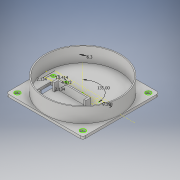
# Autodesk Inventor part: Bottom Sensor Base v1.3
Saved by Autodesk Inventor 2019 (Build 230136000, 136)
## iProperties
Created: 2020-01-12
Part Number: Bottom Sensor Base v1.3
Material: Generic
Document SubType Name: Modeling
Designer: Obscure_Decision
Density: 1 g/cm^3
Appearance: Default
Author: Obscure_Decision
Autodesk Inventor part; units mm, degrees
ref_plane "YZ Plane" through (0, 0, 0) normal (1, 0, 0) x (0, 1, 0)
ref_plane "XZ Plane" through (0, 0, 0) normal (0, 1, 0) x (-1, 0, 0)
ref_plane "XY Plane" through (0, 0, 0) normal (0, 0, 1) x (1, 0, 0)
sketch "Bottom" plane through (0, 0, 0) normal (0, 0, 1) x (1, 0, 0)
  line L0 (0, 0) -> (88.9, 0)
  line L1 (88.9, 0) -> (88.9, -3.0988)
  line L2 (88.9, -3.0988) -> (0, -3.0988)
  line L3 (0, -3.0988) -> (0, 0)
  line L4 (44.45, -3.0988) -> (44.45, 0)
  line L5 (44.45, 0) -> (90.932, 0)
  line L6 (44.45, 0) -> (90.932, 0)
  line L7 (90.932, 0) -> (90.932, -3.0988)
  line L8 (90.932, -3.0988) -> (44.45, -3.0988)
  line L9 (44.45, -3.0988) -> (44.45, 0)
  line L10 (44.45, 0) -> (-2.032, 0)
  line L11 (-2.032, 0) -> (-2.032, -3.0988)
  line L12 (-2.032, -3.0988) -> (44.45, -3.0988)
  line L13 (44.45, -3.0988) -> (44.45, 0)
  dimension "d0" = 88.9
  dimension "d1" = 3.0988
  dimension "d3" = 46.482
  dimension "d4" = 46.482
  constraints: 28 end point, 6 parallel, 4 horizontal, 3 perpendicular, 2 midpoint
  measures "d0" distance of L1.end L2.end
  measures "d1" distance of L0.end L1.end
  measures "d3" distance of L7.end L8.end
  measures "d4" distance of L11.end L12.end
revolve "Bottom Base" add sketch "Bottom" angle 360 about axis through (44.45, -3.0988, 0) along (0, 1, 0)
sketch "Outer Wall Circles" plane through (44.45, 0, 0) normal (0, 1, 0) x (1, 0, 0)
  circle A0 centre (0, 0) radius 44.45
  circle A1 centre (0, 0) radius 45.72
  point P0 (-44.45, 0)
  dimension "d6" = 88.9
  dimension "d77" = 91.44
  constraints: 2 centre point, 1 coincident
  measures "d6" diameter of A0
  measures "d77" diameter of A1
extrude "Outer Wall Extr" add sketch "Outer Wall Circles" along normal blind 17.78
sketch "Mount Square" plane through (44.45, -3.0988, 0) normal (0, -1, 0) x (1, 0, 0)
  circle A0 centre (0, 0) radius 46.482
  line L0 (43.307, -46.482) -> (-43.307, -46.482)
  line L1 (-46.482, -43.307) -> (-46.482, 43.307)
  line L2 (-43.307, 46.482) -> (43.307, 46.482)
  line L3 (46.482, 43.307) -> (46.482, -43.307)
  line L4 (46.482, -46.482) -> (-46.482, 46.482) construction
  line L5 (-46.482, -46.482) -> (46.482, 46.482) construction
  arc A1 (-46.482, -43.307) -> (-43.307, -46.482) centre (-43.307, -43.307) ccw
  arc A2 (43.307, -46.482) -> (46.482, -43.307) centre (43.307, -43.307) ccw
  arc A3 (46.482, 43.307) -> (43.307, 46.482) centre (43.307, 43.307) ccw
  arc A4 (-43.307, 46.482) -> (-46.482, 43.307) centre (-43.307, 43.307) ccw
  point P0 (-44.45, 0)
  dimension "d30" = 3.175
  constraints: 12 end point, 8 point on circle, 8 point on line, 8 tangent, 5 centre point, 3 equal radius, 2 midpoint, 2 parallel, 1 horizontal, 1 perpendicular
  measures "d30" radius of A1
extrude "Base Mount" add sketch "Mount Square" against normal blind 3.0988 contours L3 A2 L0 A0 | A0 L2 A3 L3 | A0 L1 A4 L2 | L0 A1 L1 A0
sketch "Silicon Circles" plane through (1.143, -3.0988, 46.482) normal (0, -1, 0) x (1, 0, 0)
  line L0 (89.789, -3.175) -> (89.789, -89.789) projected
  circle A0 centre (43.1405, -46.482) radius 44.45
  circle A1 centre (43.1405, -46.482) radius 43.18
  point P0 (-1.143, -46.482)
  dimension "d37" = 88.9
  dimension "d38" = 86.36
  constraints: 2 centre point, 1 coincident
  measures "d37" diameter of A0
  measures "d38" diameter of A1
extrude "Silicon Hole" cut sketch "Silicon Circles" against normal blind 1.0414
sketch "HX711-MCU Design" plane through (44.45, 0, 0) normal (0, 1, 0) x (1, 0, 0)
  line L0 (0, 0) -> (-44.45, 0) construction
  line L1 (-23.3172, -8.1296) -> (-30.9372, -8.1296)
  line L2 (-30.9372, -8.1296) -> (-30.9372, -25.9096)
  line L3 (-30.9372, -25.9096) -> (-23.3172, -25.9096)
  line L4 (-23.3172, -25.9096) -> (-23.3172, -8.1296)
  dimension "d57" = 7.62
  dimension "d58" = 17.78
  constraints: 10 end point, 2 horizontal, 2 parallel, 1 perpendicular
  measures "d57" distance of L3.end L2.end
  measures "d58" distance of L1.end L2.end
extrude "HX711 - MCU Hole" cut sketch "HX711-MCU Design" against normal blind 3.1242
sketch "hx711 mount" plane through (44.45, 0, 0) normal (0, 1, 0) x (1, 0, 0)
  line L0 (20.11, -38.7522) -> (-20.11, -38.7522)
  line L1 (-20.11, -38.7522) -> (-20.11, -32.6906)
  line L2 (-20.11, -10.3514) -> (20.11, -10.3514)
  line L3 (20.11, -10.3514) -> (20.11, -16.413)
  line L4 (17.765, -37.0963) -> (-17.765, -12.0073) construction
  line L5 (-17.765, -37.0963) -> (17.765, -12.0073) construction
  line L6 (17.765, -37.0963) -> (-17.765, -37.0963)
  line L7 (-17.765, -37.0963) -> (-17.765, -32.6906)
  line L8 (-17.765, -12.0073) -> (17.765, -12.0073)
  line L9 (17.765, -12.0073) -> (17.765, -16.413)
  line L10 (17.765, -37.0963) -> (-17.765, -12.0073) construction
  line L11 (-17.765, -37.0963) -> (-11.5259, -32.6906) construction
  line L12 (0, -24.5518) -> (17.765, -24.5518) construction
  line L13 (-17.765, -32.6906) -> (-20.11, -32.6906)
  line L14 (-11.5259, -32.6906) -> (17.765, -12.0073) construction
  line L15 (-20.11, -16.413) -> (-17.765, -16.413)
  line L16 (17.765, -32.6906) -> (20.11, -32.6906)
  line L17 (17.765, -16.413) -> (20.11, -16.413)
  line L18 (-17.765, -12.0073) -> (17.765, -12.0073)
  line L19 (17.765, -12.0073) -> (17.765, -16.413)
  line L20 (17.765, -37.0963) -> (-17.765, -37.0963)
  line L21 (-17.765, -37.0963) -> (-17.765, -32.6906)
  line L22 (-20.11, -38.7522) -> (20.11, -38.7522)
  line L23 (20.11, -38.7522) -> (20.11, -32.6906)
  line L24 (20.11, -10.3514) -> (-20.11, -10.3514)
  line L25 (-20.11, -10.3514) -> (-20.11, -16.413)
  line L26 (-17.765, -16.413) -> (-17.765, -12.0073)
  line L27 (-20.11, -16.413) -> (-20.11, -10.3514)
  line L28 (17.765, -32.6906) -> (17.765, -37.0963)
  line L29 (17.765, -32.6906) -> (17.765, -37.0963)
  line L30 (20.11, -32.6906) -> (20.11, -38.7522)
  line L31 (20.11, -16.413) -> (20.11, -10.3514)
  line L32 (-20.11, -32.6906) -> (-20.11, -38.7522)
  line L33 (-17.765, -16.413) -> (-17.765, -12.0073)
  point P0 (-44.45, 0)
  point P1 (-17.765, -32.6906)
  constraints: 68 end point, 20 parallel, 14 perpendicular, 4 horizontal, 4 point on line, 3 midpoint, 1 symmetric about line
sketch "Bottom Circles" plane through (44.45, 0, 0) normal (0, 1, 0) x (1, 0, 0)
  line L0 (-16.2451, -6.4091) -> (-16.2451, 6.2909) construction
  line L1 (-22.9507, -0.0591) -> (-16.2451, -0.0591) construction
  line L2 (-22.9507, -0.0591) -> (-18.3787, -0.0591) construction
  circle A0 centre (-20.6647, -0.0591) radius 2.286
  line L3 (-33.3647, -0.0591) -> (-22.9507, -0.0591) construction
  line L4 (-33.3647, -0.0591) -> (-40.0703, -0.0591) construction
  line L5 (-40.0703, 6.2909) -> (-40.0703, -6.4091) construction
  line L6 (-16.2451, -6.4091) -> (-40.0703, -6.4091) construction
  line L7 (-40.0703, -6.4091) -> (-40.0703, 6.2909) construction
  line L8 (-40.0703, 6.2909) -> (-16.2451, 6.2909) construction
  line L9 (-16.2451, 6.2909) -> (-16.2451, -6.4091) construction
  line L10 (-28.1577, -0.0591) -> (-28.1577, -6.4091) construction
  line L11 (-40.0703, -6.4091) -> (-16.2451, -6.4091) construction
  circle A1 centre (-35.6507, -0.0591) radius 2.286
  line L12 (0, 0) -> (0, 6.2909) construction
  line L13 (0, 0) -> (-45.3601, 45.3601) construction
  line L14 (0, 0) -> (64.1489, 0) construction
  circle A2 centre (-39.6699, 39.6699) radius 3.15
  circle A3 centre (39.6699, 39.6699) radius 3.15
  line L15 (0, 0) -> (6.017, 0) construction
  circle A4 centre (-39.6699, -39.6699) radius 3.15
  circle A5 centre (39.6699, -39.6699) radius 3.15
  point P0 (-44.45, 0)
  dimension "d103" = 4.572
  dimension "d104" = 10.414
  dimension "d105" = 2.1336
  dimension "d106" = 2.1336
  dimension "d113" = 135
  dimension "d114" = 6.3
  constraints: 32 end point, 5 centre point, 5 midpoint, 4 symmetric about line, 3 horizontal, 2 parallel, 2 perpendicular, 2 point on line, 1 equal length, 1 horizontal alignment, 1 vertical, 6 other
  measures "d103" distance of L1.start L2.end
  measures "d104" distance of L3.start L1.start
  measures "d105" distance from line of L2.end L0
  measures "d106" distance edge to line of A1 L5
  measures "d113" angle of L14 L13
  measures "d114" diameter of A2
extrude "Bottom Holes" cut sketch "Bottom Circles" against normal blind 4 contours A0 | A1
sketch "Top Shadow" plane through (44.45, 0, 0) normal (0, 1, 0) x (1, 0, 0)
  line L0 (27.4022, -6.3354) -> (27.4022, 6.3646) construction
  circle A0 centre (34.8952, 0.0146) radius 2.794 construction
  circle A1 centre (19.9092, 0.0146) radius 2.794 construction
  line L1 (22.7032, 0.0146) -> (32.1012, 0.0146) construction
  line L2 (14.7022, -6.3354) -> (40.1022, -6.3354) construction
  line L3 (40.1022, -6.3354) -> (40.1022, 6.3646) construction
  line L4 (40.1022, 6.3646) -> (14.7022, 6.3646) construction
  line L5 (14.7022, 6.3646) -> (14.7022, -6.3354) construction
  line L6 (14.7022, -6.3354) -> (40.1022, 6.3646) construction
  line L7 (40.1022, -6.3354) -> (14.7022, 6.3646) construction
  line L8 (40.065, -6.3646) -> (-40.065, -6.3646) construction
  line L9 (-40.065, -6.3646) -> (-40.065, 6.3646) construction
  line L10 (-40.065, 6.3646) -> (40.065, 6.3646) construction
  line L11 (40.065, 6.3646) -> (40.065, -6.3646) construction
  line L12 (40.065, -6.3646) -> (-40.065, 6.3646) construction
  line L13 (-40.065, -6.3646) -> (40.065, 6.3646) construction
  point P0 (27.4022, 0.0146)
  point P1 (0, 0)
  dimension "d109" = 9.398
  constraints: 28 end point, 5 midpoint, 4 parallel, 3 horizontal, 2 horizontal alignment, 2 perpendicular, 1 symmetric about line, 1 vertical, 4 other
  measures "d109" distance of L1.start L1.end
extrude "Base to Rail Mount" cut sketch "Bottom Circles" against normal blind 4 contours A2 | A3 | A4 | A5
extrude "hx711 walls" add sketch "hx711 mount" along normal blind 10
body "Solid1"
